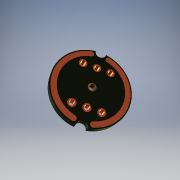
# Autodesk Inventor part: INMP441 MEMS I2S MICROPHONE PCB
Saved by Autodesk Inventor 2016 SP2 (Build 200237200, 237)
## iProperties
Created: 2023-04-15
Part Number: INMP441 MEMS I2S MICROPHONE PCB
Material: Generic
Document SubType Name: Modeling
Designer: Mark
Density: 1 g/cm^3
Appearance: Dark Olive
Author: Mark
Autodesk Inventor part; units mm, degrees
ref_plane "YZ Plane" through (0, 0, 0) normal (1, 0, 0) x (0, 1, 0)
ref_plane "XZ Plane" through (0, 0, 0) normal (0, 1, 0) x (-1, 0, 0)
ref_plane "XY Plane" through (0, 0, 0) normal (0, 0, 1) x (1, 0, 0)
sketch "Sketch1" plane through (0, 0, 0) normal (0, 1, 0) x (-1, 0, 0)
  circle A0 centre (2.5, -3.75) radius 0.5
  line L0 (4.5047, -13.3747) -> (-4.6881, -13.3747) construction
  circle A1 centre (0, -3.75) radius 0.5
  circle A2 centre (-2.5, -3.75) radius 0.5
  circle A3 centre (2.5, 3.75) radius 0.5
  circle A4 centre (0, 3.75) radius 0.5
  circle A5 centre (-2.5, 3.75) radius 0.5
  arc A6 (-0.9974, 6.9286) -> (0.9974, 6.9286) centre (0, 7) ccw
  arc A7 (0.9974, -6.9286) -> (-0.9974, -6.9286) centre (0, -7) ccw
  arc A8 (-0.9974, 6.9286) -> (-0.9974, -6.9286) centre (0, 0) ccw
  arc A9 (0.9974, -6.9286) -> (0.9974, 6.9286) centre (0, 0) ccw
  arc A10 (-0.9974, 6.9286) -> (-6.9286, 0.9974) centre (0, 0) ccw
  dimension "d3" = 1
  dimension "d6" = 2.5
  dimension "d16" = 1
  dimension "d17" = 2.5
  constraints: 11 centre point, 10 point on circle, 2 end point, 2 horizontal, 1 coincident
  measures "d3" diameter of A0
  measures "d6" distance of A0.centre A1.centre
  measures "d16" diameter of A3
  measures "d17" distance of A3.centre A4.centre
extrude "Extrusion1" add sketch "Sketch1" along normal mid plane 1.4
sketch "Sketch2" plane through (0, -0.7, 0) normal (0, -1, 0) x (1, 0, 0)
  circle A0 centre (0, 0) radius 0.6
  dimension "d20" = 1.2
  constraints: 1 centre point, 1 coincident
  measures "d20" diameter of A0
extrude "Extrusion2" cut sketch "Sketch2" against normal through all
sketch "Sketch3" plane through (0, 0.7, 0) normal (0, 1, 0) x (1, 0, 0)
  circle A0 centre (-2.5, 3.75) radius 0.5 projected
  circle A1 centre (-2.5, 3.75) radius 0.75
  point P0 (0, 0)
  dimension "d23" = 1.5
  constraints: 1 centre point, 1 coincident
  measures "d23" diameter of A1
extrude "Extrusion3" add sketch "Sketch3" along normal blind 0.005 separate body
pattern_linear "Rectangular Pattern1" count 3 spacing 2.5 along (1, 0, 0) count 2 spacing 7.5 along (0, 0, 1) of "Extrusion3" bodies 2
mirror "Mirror1" about plane through (0, 0, 0) normal (0, 1, 0) of "Extrusion3", "Rectangular Pattern1" bodies 2
sketch "Sketch4" plane through (0, 0.7, 0) normal (0, 1, 0) x (1, 0, 0)
  arc A0 (0.9974, -6.9286) -> (0.9974, 6.9286) centre (0, 0) ccw projected
  arc A1 (-0.9974, 6.9286) -> (-0.9974, -6.9286) centre (0, 0) ccw projected
  arc A2 (-1.7147, 6.5735) -> (-1.7147, -6.5735) centre (0, 0) ccw
  line L0 (-9.685, 0) -> (-13.1898, 0) construction
  arc A3 (-1.4623, 5.6059) -> (-1.4623, -5.6059) centre (0, 0) ccw
  arc A4 (-1.7147, -6.5735) -> (-1.4623, -5.6059) centre (-1.5885, -6.0897) ccw
  line L1 (0, 11.7896) -> (0, 9.2828) construction
  arc A5 (-1.4623, 5.6059) -> (-1.7147, 6.5735) centre (-1.5885, 6.0897) ccw
  point P0 (-6.9286, 0.9974)
  point P1 (6.9286, -0.9974)
  dimension "d32" = 1
  constraints: 8 point on circle, 4 centre point, 4 end point, 1 horizontal, 1 vertical
  measures "d32" radial gap between concentric circles of A2 A3
extrude "Extrusion4" add sketch "Sketch4" along normal blind 0.005 separate body
mirror "Mirror2" about plane through (0, 0, 0) normal (1, 0, 0) of "Extrusion4" bodies 3
mirror "Mirror3" about plane through (0, 0, 0) normal (0, 1, 0) of "Extrusion4", "Mirror2" bodies 3
sketch "Sketch5" plane through (0, -0.7, 0) normal (0, -1, 0) x (1, 0, 0)
  circle A0 centre (0, 0) radius 0.6 projected
  circle A1 centre (0, 0) radius 0.75
  dimension "d35" = 1.5
  constraints: 1 centre point, 1 coincident
  measures "d35" diameter of A1
extrude "Extrusion5" add sketch "Sketch5" along normal blind 0.005 separate body
body "Solid1"
body "Solid2"
body "Solid3"
body "Solid4"
